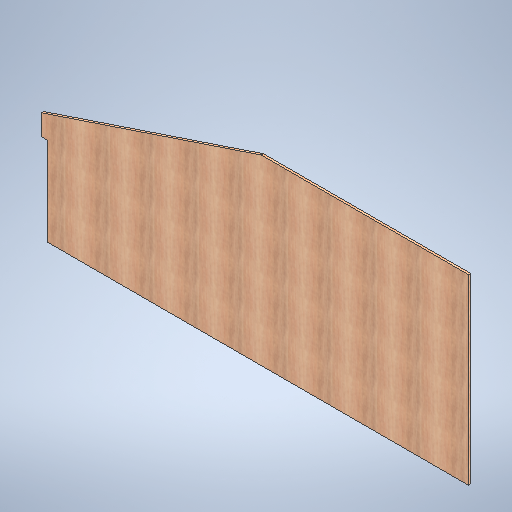
# Autodesk Inventor part: OSB_For_Side_And_Back
Saved by Autodesk Inventor 2025.1 (Build 291241020, 241B)
## iProperties
Created: 2024-09-19
Part Number: OSB_For_Side_And_Back
Material: Wood (Birch)
Document SubType Name: Modeling
Designer: Tom
Density: 0.55 g/cm^3
Appearance: Birch - Natural Polished
Author: Tom
Autodesk Inventor part; units mm, degrees
ref_plane "YZ Plane" through (0, 0, 0) normal (1, 0, 0) x (0, 1, 0)
ref_plane "XZ Plane" through (0, 0, 0) normal (0, 1, 0) x (-1, 0, 0)
ref_plane "XY Plane" through (0, 0, 0) normal (0, 0, 1) x (1, 0, 0)
sketch "Sketch1" plane through (0, 0, 0) normal (0, 0, 1) x (1, 0, 0)
  line L0 (0, 0) -> (0, 617.0676)
  line L1 (0, 0) -> (1219.2, 0)
  line L2 (0, 617.0676) -> (3365.5, 1739.9922)
  line L3 (12.7, 621.3051) -> (12.7, 0)
  line L4 (3365.5, 1739.9922) -> (3365.5, 1592.7212)
  line L5 (3365.5, 1592.7212) -> (101.6, 503.6962)
  line L6 (101.6, 503.6962) -> (12.7, 503.6962)
  line L7 (1219.2, 0) -> (1219.2, 1023.8629)
  line L8 (0, 617.0676) -> (-35.0901, 605.3595)
  line L9 (-35.0901, 605.3595) -> (-35.0901, 503.6962)
  line L10 (-35.0901, 503.6962) -> (0, 503.6962)
  line L11 (-35.0901, 622.0949) -> (1219.2, 1040.5983)
  line L12 (1219.2, 1040.5983) -> (1219.2, 1023.8629)
  line L13 (1219.2, 1040.5983) -> (2401.8875, 1040.5983)
  line L14 (2401.8875, 1040.5983) -> (2401.8875, 0)
  line L15 (2401.8875, 0) -> (1219.2, 0)
  line L16 (-35.0901, 605.3595) -> (-35.0901, 622.0949)
  point P0 (1219.2, 876.5919)
  point P1 (1710.7411, 1040.5983)
  point P2 (1269.3573, 1040.5983)
  dimension "d1" = 617.0676
  dimension "d3" = 12.7
  dimension "d4" = 3352.8
  dimension "d6" = 139.7
  dimension "d8" = 88.9
  dimension "d9" = 1089.025
  dimension "d12" = 47.7901
  dimension "d14" = 15.875
  dimension "d16" = 1219.2
  dimension "d18" = 2436.9776
  constraints: 34 end point, 8 vertical, 5 horizontal, 5 point on line, 2 collinear, 2 parallel
  measures "d1" distance of L0.start L0.end
  measures "d3" distance between parallel lines of L3 L0
  measures "d4" distance from line of L3 L2.end
  measures "d6" distance between parallel lines of L2 L5
  measures "d8" horizontal distance of L3.start L5.end
  measures "d9" vertical distance of L4.end L5.end
  measures "d12" distance between parallel lines of L9 L3
  measures "d14" distance between parallel lines of L2 L11
  measures "d16" distance of L0.start L1.end
  measures "d18" distance between parallel lines of L14 L9
extrude "Extrusion1" add sketch "Sketch1" along normal blind 12.7 contours L0 L2 L3 L1 | L10 L9 L8 L0 | L3 L6 L5 L7 L1 | L8 L16 L11 L12 L2 | L7 L5 L13 L14 L15 | L3 L2 L7 L5 L6 | L7 L2 L13 L5 | L12 L13 L2
body "Solid1"
